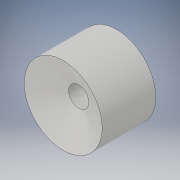
# Autodesk Inventor part: 85mmWheel
Saved by Autodesk Inventor 2018 (Build 220112000, 112)
## iProperties
Created: 2019-06-09
Part Number: 85mmWheel
Material: Generic
Document SubType Name: Modeling
Designer: anirudh
Density: 1 g/cm^3
Appearance: Default
Author: anirudh
Autodesk Inventor part; units mm, degrees
ref_plane "YZ Plane" through (0, 0, 0) normal (1, 0, 0) x (0, 1, 0)
ref_plane "XZ Plane" through (0, 0, 0) normal (0, 1, 0) x (-1, 0, 0)
ref_plane "XY Plane" through (0, 0, 0) normal (0, 0, 1) x (1, 0, 0)
sketch "Sketch2" plane through (0, 0, 0) normal (1, 0, 0) x (0, 1, 0)
  line L0 (85, 29.25) -> (85, -29.25)
  line L1 (53.5, 0) -> (53.5, 10)
  line L2 (53.5, 0) -> (53.5, -10)
  line L3 (42.5, 0) -> (42.5, -56.6203)
  line L4 (53.5, 10) -> (53.5, 12.3241)
  line L5 (53.5, 12.3241) -> (85, 29.25)
  line L6 (53.5, -10) -> (53.5, -12.3241)
  line L7 (53.5, -12.3241) -> (85, -29.25)
  point P0 (0, 0)
  dimension "d6" = 11
  dimension "d7" = 10
  dimension "d10" = 2.3241
  dimension "d11" = 2.3241
  constraints: 16 end point, 3 vertical, 1 point on line
  measures "d6" distance of L3.start L1.start
  measures "d7" distance of L1.start L1.end
  measures "d10" distance of L1.end L4.end
  measures "d11" distance of L2.end L6.end
revolve "Revolution1" add sketch "Sketch2" angle 360 about axis through (0, 42.5, 0) along (0, 0, -1)
body "Solid1"
